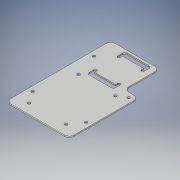
# Autodesk Inventor part: Tier1Plate
Saved by Autodesk Inventor 2018 (Build 220112000, 112)
## iProperties
Created: 2019-03-24
Part Number: Tier1Plate
Material: Generic
Document SubType Name: Modeling
Designer: anirudh
Density: 1 g/cm^3
Appearance: Default
Author: anirudh
Autodesk Inventor part; units mm, degrees
ref_plane "YZ Plane" through (0, 0, 0) normal (1, 0, 0) x (0, 1, 0)
ref_plane "XZ Plane" through (0, 0, 0) normal (0, 1, 0) x (-1, 0, 0)
ref_plane "XY Plane" through (0, 0, 0) normal (0, 0, 1) x (1, 0, 0)
sketch "Sketch1" plane through (0, 0, 0) normal (0, 1, 0) x (-1, 0, 0)
  line L0 (53.6232, -76.2) -> (19.5232, -76.2)
  line L1 (50.0232, -82.55) -> (23.1232, -82.55)
  line L2 (23.1232, -118.55) -> (50.0232, -118.55)
  arc A0 (50.0232, -85.3) -> (53.6232, -85.3) centre (51.8232, -85.3) ccw
  arc A1 (53.6232, -115.8) -> (50.0232, -115.8) centre (51.8232, -115.8) ccw
  arc A2 (19.5232, -85.3) -> (23.1232, -85.3) centre (21.3232, -85.3) ccw
  arc A3 (23.1232, -115.8) -> (19.5232, -115.8) centre (21.3232, -115.8) ccw
  circle A4 centre (58.1025, -6.35) radius 1.8
  circle A5 centre (58.1025, -69.85) radius 1.8
  circle A6 centre (10.4775, -6.35) radius 1.8
  circle A7 centre (10.4775, -69.85) radius 1.8
  line L3 (74.93, 6.35) -> (-6.35, 6.35)
  line L4 (74.93, -95.25) -> (74.93, 6.35)
  line L5 (-6.35, 6.35) -> (-6.35, -82.55)
  line L6 (12.23, -124.9) -> (12.23, -128.075)
  line L7 (12.23, -88.9) -> (12.23, -128.075)
  line L8 (74.93, -128.075) -> (74.93, -95.25)
  line L9 (18.58, -128.075) -> (12.23, -128.075)
  line L10 (12.23, -128.075) -> (74.93, -128.075)
  line L11 (12.23, -88.9) -> (12.23, -82.55)
  line L12 (12.23, -82.55) -> (-6.35, -82.55)
  line L13 (53.6232, -124.9) -> (19.5232, -124.9)
  line L14 (19.5232, -85.3) -> (19.5232, -82.55)
  line L15 (23.1232, -85.3) -> (23.1232, -82.55)
  line L16 (53.6232, -85.3) -> (53.6232, -82.55)
  line L17 (50.0232, -85.3) -> (50.0232, -82.55)
  line L18 (53.6232, -115.8) -> (53.6232, -118.55)
  line L19 (50.0232, -115.8) -> (50.0232, -118.55)
  line L20 (19.5232, -115.8) -> (19.5232, -124.9)
  line L21 (23.1232, -115.8) -> (23.1232, -118.55)
  line L22 (19.5232, -85.3) -> (19.5232, -76.2)
  line L23 (53.6232, -85.3) -> (53.6232, -76.2)
  line L24 (53.6232, -115.8) -> (53.6232, -124.9)
  line L25 (74.93, -128.075) -> (68.58, -128.075)
  circle A8 centre (0, -76.2) radius 1.8
  circle A9 centre (68.58, -21.4884) radius 1.8
  circle A10 centre (68.58, -100.2366) radius 1.8
  circle A11 centre (0, -21.4884) radius 1.8
  point P0 (0, 0)
  dimension "d13" = 3.6
  dimension "d14" = 3.6
  dimension "d15" = 3.6
  dimension "d16" = 3.6
  dimension "d22" = 3.6
  dimension "d23" = 3.6
  dimension "d24" = 3.6
  dimension "d25" = 3.6
  dimension "d47" = 3.6
  dimension "d56" = 3.6
  dimension "d57" = 3.6
  dimension "d58" = 3.6
  constraints: 52 end point, 12 centre point, 12 perpendicular, 8 point on circle, 7 point on line, 6 tangent, 2 horizontal, 2 vertical, 1 collinear, 1 parallel
  measures "d13" diameter of A0
  measures "d14" diameter of A1
  measures "d15" diameter of A2
  measures "d16" diameter of A3
  measures "d22" diameter of A4
  measures "d23" diameter of A5
  measures "d24" diameter of A6
  measures "d25" diameter of A7
  measures "d47" diameter of A8
  measures "d56" diameter of A9
  measures "d57" diameter of A10
  measures "d58" diameter of A11
extrude "Extrusion2" add sketch "Sketch1" along normal blind 1.5875
fillet "Fillet3" radius 6.35 6 edges at (6.35, 0.7937, -82.55) (6.35, 0.7937, 6.35) (-12.23, 0.7937, -82.55) (-12.23, 0.7937, -128.075) (-74.93, 0.7937, -128.075) (-74.93, 0.7937, 6.35)
fillet "Fillet4" radius 3.175 4 edges at (-19.5232, 0.7937, -124.9) (-53.6232, 0.7937, -124.9) (-19.5232, 0.7937, -76.2) (-53.6232, 0.7937, -76.2)
sketch "Sketch2" plane through (0, 1.5875, 0) normal (0, 1, 0) x (1, 0, 0)
  line L0 (-23.1232, 82.55) -> (-50.0232, 82.55) projected
  line L1 (-50.0232, 82.55) -> (-53.6232, 82.55)
  line L2 (-53.6232, 85.3) -> (-53.6232, 79.375) projected
  line L3 (-23.1232, 85.3) -> (-23.1232, 82.55) projected
  line L4 (-23.1232, 82.55) -> (-19.5232, 82.55)
  line L5 (-19.5232, 79.375) -> (-19.5232, 85.3) projected
  line L6 (-50.0232, 118.55) -> (-23.1232, 118.55) projected
  line L7 (-23.1232, 118.55) -> (-19.5232, 118.55)
  line L8 (-19.5232, 121.725) -> (-19.5232, 115.8) projected
  line L9 (-50.0232, 115.8) -> (-50.0232, 118.55) projected
  line L10 (-50.0232, 118.55) -> (-53.6232, 118.55)
  line L11 (-53.6232, 115.8) -> (-53.6232, 121.725) projected
  arc A0 (-53.6232, 115.8) -> (-50.0232, 115.8) centre (-51.8232, 115.8) ccw projected
  line L12 (-50.0232, 115.8) -> (-50.0232, 118.55)
  line L13 (-53.6232, 118.55) -> (-53.6232, 115.8)
  arc A1 (-53.6232, 115.8) -> (-50.0232, 115.8) centre (-51.8232, 115.8) ccw
  arc A2 (-50.0232, 85.3) -> (-53.6232, 85.3) centre (-51.8232, 85.3) ccw projected
  arc A3 (-50.0232, 85.3) -> (-53.6232, 85.3) centre (-51.8232, 85.3) ccw
  arc A4 (-19.5232, 85.3) -> (-23.1232, 85.3) centre (-21.3232, 85.3) ccw projected
  arc A5 (-19.5232, 85.3) -> (-23.1232, 85.3) centre (-21.3232, 85.3) ccw
  arc A6 (-23.1232, 115.8) -> (-19.5232, 115.8) centre (-21.3232, 115.8) ccw projected
  arc A7 (-23.1232, 115.8) -> (-19.5232, 115.8) centre (-21.3232, 115.8) ccw
  line L14 (-19.5232, 115.8) -> (-19.5232, 118.55)
  line L15 (-23.1232, 115.8) -> (-23.1232, 118.55)
  line L16 (-19.5232, 82.55) -> (-19.5232, 85.3)
  line L17 (-23.1232, 85.3) -> (-23.1232, 82.55)
  line L18 (-50.0232, 82.55) -> (-50.0232, 85.3) projected
  line L19 (-50.0232, 85.3) -> (-50.0232, 82.55)
  line L20 (-53.6232, 85.3) -> (-53.6232, 82.55)
  point P0 (0, 0)
  constraints: 24 end point, 8 point on circle, 6 point on line, 5 tangent, 4 centre point, 4 coincident, 3 parallel, 3 vertical, 2 perpendicular, 1 collinear, 1 horizontal
body "Solid2"
